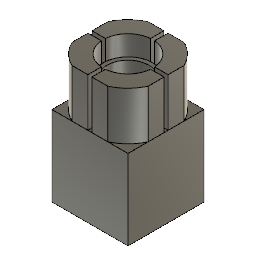
rubic_center_holder v1 (Autodesk Fusion 360 design; units mm, degrees)
Autodesk Fusion 360 part; units mm, degrees
note: some values were not read from the file. Set by a fixed rule: which sketch regions a step uses.
sketch "Sketch1" plane through (0, 0, 0) normal (0, 0, 1) x (1, 0, 0)
  circle A0 centre (0, 0) radius 5.15
  circle A1 centre (0, 0) radius 6.15
  line L0 (9.5, 9.5) -> (-9.5, 9.5)
  line L1 (-9.5, 9.5) -> (-9.5, -9.5)
  line L2 (-9.5, -9.5) -> (9.5, -9.5)
  line L3 (9.5, -9.5) -> (9.5, 9.5)
  line L4 (9.5, 9.5) -> (-9.5, -9.5) construction
  line L5 (-9.5, 9.5) -> (9.5, -9.5) construction
  line L6 (-7.4246, 7.4246) -> (7.4246, -7.4246) construction
  arc A2 (-4.4721, 9.5) -> (-9.5, 4.4721) centre (0, 0) ccw
  line L7 (-2.75, 0) -> (2.25, 0) construction
  line L8 (2.25, 1.5811) -> (2.25, -1.5811)
  arc A3 (2.25, 1.5811) -> (2.25, -1.5811) centre (0, 0) ccw
  arc A4 (-9.5, -4.4721) -> (-4.4721, -9.5) centre (0, 0) ccw
  arc A5 (4.4721, -9.5) -> (9.5, -4.4721) centre (0, 0) ccw
  arc A6 (9.5, 4.4721) -> (4.4721, 9.5) centre (0, 0) ccw
  line L9 (-0.5, 9.5) -> (0.5, 9.5) construction
  line L10 (0.5, 9.5) -> (0.5, -9.5)
  line L11 (0.5, -9.5) -> (-0.5, -9.5) construction
  line L12 (-0.5, -9.5) -> (-0.5, 9.5)
  line L13 (-0.5, 9.5) -> (0.5, -9.5) construction
  line L14 (0.5, 9.5) -> (-0.5, -9.5) construction
  line L15 (-9.5, 0.5) -> (9.5, 0.5)
  line L16 (9.5, 0.5) -> (9.5, -0.5) construction
  line L17 (9.5, -0.5) -> (-9.5, -0.5)
  line L18 (-9.5, -0.5) -> (-9.5, 0.5) construction
  line L19 (-9.5, 0.5) -> (9.5, -0.5) construction
  line L20 (9.5, 0.5) -> (-9.5, -0.5) construction
  dimension "d1" = 10.3
  dimension "d2" = 1
  dimension "d3" = 19
  dimension "d4" = 19
  dimension "d5" = 21
  dimension "d6" = 5.5
  dimension "d7" = 5
  dimension "d9" = 360
  dimension "d10" = 1
  dimension "d11" = 19
  dimension "d12" = 1
  constraint coincident A0.centre A1.centre
  constraint horizontal L0
  constraint perpendicular L0 L1
  constraint parallel L0 L2
  constraint parallel L1 L3
  constraint coincident L4 A0.centre
  constraint coincident L5 A0.centre
  constraint parallel L5 L6
  constraint midpoint A0.centre L6
  constraint concentric A0 A2
  constraint coincident L6.start A2
  constraint coincident L0 A2.start
  constraint coincident L1 A2.end
  constraint coincident L7.start A3
  constraint horizontal L7
  constraint vertical L8
  constraint midpoint L7.end L8
  constraint horizontal L9
  constraint perpendicular L9 L10
  constraint parallel L9 L11
  constraint parallel L10 L12
  constraint coincident L13 A0.centre
  constraint coincident L14 A0.centre
  constraint horizontal L15
  constraint perpendicular L15 L16
  constraint parallel L15 L17
  constraint parallel L16 L18
  constraint coincident L19 A0.centre
  constraint coincident L20 A0.centre
  measures "d1" diameter of A0
  measures "d3" distance of L1.end L2.end
  measures "d4" distance of L0.end L1.end
  measures "d5" distance of L6.start L6.end
  measures "d6" diameter of A3
  measures "d7" distance of L7.start L7.end
  measures "d10" distance of L10.end L11.end
  measures "d11" distance of L16.end L17.end
  measures "d12" distance of L15.end L16.end
extrude "Extrude1" add sketch "Sketch1" along normal blind 12 contours A1 L0 L3 A6 L10 L15 | A1 L2 L3 A5 L10 L17 | A1 L0 L1 A2 L12 L15 | A1 L1 L2 A4 L12 L17 makes body 1 at (6.0994, 0.787, 4) makes body 2 at (-1.0723, -6.0558, 8) makes body 3 at (-3.922, 4.7372, 8) makes body 4 at (3.922, -4.7372, 8)
extrude "Extrude2" add sketch "Sketch1" along normal blind 7 contours A0 A1 L10 L15 | A0 A1 L10 L17 | A0 A1 L10 L12 | A0 A1 L10 L12 | A0 A1 L12 L15 | A0 A1 L12 L17 | A0 A1 L15 L17 picked at (-5.4675, -0.389) bodies 1 2 3 4
extrude "Extrude3" add sketch "Sketch1" against normal blind 20 separate body makes body 5
sketch "Sketch2" plane through (0, 0, -20) normal (0, 0, -1) x (1, 0, 0)
  line L0 (9.5, -9.5) -> (9.5, 9.5)
  line L1 (9.5, 9.5) -> (-9.5, 9.5)
  line L2 (-9.5, 9.5) -> (-9.5, -9.5)
  line L3 (-9.5, -9.5) -> (9.5, -9.5)
  arc A0 (2.25, 1.5811) -> (2.25, -1.5811) centre (0, 0) ccw
  line L4 (2.25, -1.5811) -> (2.25, 1.5811)
extrude "Extrude4" cut sketch "Sketch2" against normal blind 15 contours A0 L4 bodies 5
